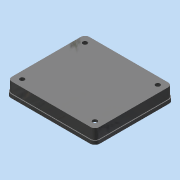
# Autodesk Inventor part: Plate
Saved by Autodesk Inventor 2012 (Build 160160000, 160)
## iProperties
Created: 2012-05-23
Part Number: Plate
Material: Default
Document SubType Name: Modeling
Designer: dgitz
Density: 1 g/cm^3
Author: dgitz
Autodesk Inventor part; units mm, degrees
ref_plane "YZ Plane" through (0, 0, 0) normal (1, 0, 0) x (0, 1, 0)
ref_plane "XZ Plane" through (0, 0, 0) normal (0, 1, 0) x (-1, 0, 0)
ref_plane "XY Plane" through (0, 0, 0) normal (0, 0, 1) x (1, 0, 0)
sketch "Sketch2" plane through (0, 0, 0) normal (0, 1, 0) x (-1, 0, 0)
  line L0 (-50.8, 50.8) -> (50.8, 50.8)
  line L1 (57.15, 44.45) -> (57.15, -44.45)
  line L2 (50.8, -50.8) -> (-50.8, -50.8)
  line L3 (-57.15, -44.45) -> (-57.15, 44.45)
  arc A0 (-50.8, 50.8) -> (-57.15, 44.45) centre (-50.8, 44.45) ccw
  arc A1 (-57.15, -44.45) -> (-50.8, -50.8) centre (-50.8, -44.45) ccw
  arc A2 (50.8, -50.8) -> (57.15, -44.45) centre (50.8, -44.45) ccw
  arc A3 (57.15, 44.45) -> (50.8, 50.8) centre (50.8, 44.45) ccw
  line L4 (50.8, 48.768) -> (-50.8, 48.768)
  arc A4 (-50.8, 48.768) -> (-55.118, 44.45) centre (-50.8, 44.45) ccw
  line L5 (-55.118, 44.45) -> (-55.118, -44.45)
  arc A5 (-55.118, -44.45) -> (-50.8, -48.768) centre (-50.8, -44.45) ccw
  line L6 (-50.8, -48.768) -> (50.8, -48.768)
  arc A6 (50.8, -48.768) -> (55.118, -44.45) centre (50.8, -44.45) ccw
  line L7 (55.118, -44.45) -> (55.118, 44.45)
  arc A7 (55.118, 44.45) -> (50.8, 48.768) centre (50.8, 44.45) ccw
  line L8 (-50.8, 44.45) -> (50.8, -44.45) construction
  point P0 (0, 0)
  point P1 (0, 0)
  point P2 (0, 0)
  dimension "d0" = 114.3
  dimension "d1" = 101.6
  dimension "d2" = 6.35
  dimension "d3" = 2.032
  constraints: 18 end point, 16 point on circle, 8 centre point, 8 tangent, 4 parallel, 3 equal radius, 2 coincident, 2 perpendicular, 1 horizontal, 1 midpoint, 7 other
  measures "d0" distance between parallel lines of L1 L3
  measures "d1" distance between parallel lines of L2 L0
  measures "d2" radius of A0
  measures "d3" distance between parallel lines of L5 L3
extrude "Extrusion1" add sketch "Sketch2" along normal blind 4.572
sketch "Sketch3" plane through (0, 4.572, 0) normal (0, 1, 0) x (1, 0, 0)
  line L0 (-55.118, -44.45) -> (-55.118, 44.45) projected
  arc A0 (-50.8, 48.768) -> (-55.118, 44.45) centre (-50.8, 44.45) ccw projected
  line L1 (-50.8, 48.768) -> (50.8, 48.768) projected
  line L2 (55.118, 44.45) -> (55.118, -44.45) projected
  line L3 (50.8, -48.768) -> (-50.8, -48.768) projected
  line L4 (-50.8, 49.784) -> (50.8, 49.784)
  line L5 (56.134, 44.45) -> (56.134, -44.45)
  line L6 (50.8, -49.784) -> (-50.8, -49.784)
  line L7 (-56.134, -44.45) -> (-56.134, 44.45)
  arc A1 (-50.8, 49.784) -> (-56.134, 44.45) centre (-50.8, 44.45) ccw
  arc A2 (-56.134, -44.45) -> (-50.8, -49.784) centre (-50.8, -44.45) ccw
  arc A3 (50.8, -49.784) -> (56.134, -44.45) centre (50.8, -44.45) ccw
  arc A4 (56.134, 44.45) -> (50.8, 49.784) centre (50.8, 44.45) ccw
  line L8 (-54.102, 44.45) -> (-54.102, -44.45)
  arc A5 (-54.102, -44.45) -> (-50.8, -47.752) centre (-50.8, -44.45) ccw
  line L9 (-50.8, -47.752) -> (50.8, -47.752)
  arc A6 (50.8, -47.752) -> (54.102, -44.45) centre (50.8, -44.45) ccw
  line L10 (54.102, -44.45) -> (54.102, 44.45)
  arc A7 (54.102, 44.45) -> (50.8, 47.752) centre (50.8, 44.45) ccw
  line L11 (50.8, 47.752) -> (-50.8, 47.752)
  arc A8 (-50.8, 47.752) -> (-54.102, 44.45) centre (-50.8, 44.45) ccw
  point P0 (0, 0)
  dimension "d7" = 1.016
  dimension "d8" = 1.016
  dimension "d9" = 1.016
  dimension "d10" = 1.016
  dimension "d11" = 2.032
  constraints: 16 end point, 16 point on circle, 8 centre point, 8 tangent, 4 parallel, 3 equal radius, 2 perpendicular, 1 concentric, 1 horizontal, 7 other
  measures "d7" distance between parallel lines of L7 L0
  measures "d8" distance between parallel lines of L4 L1
  measures "d9" distance between parallel lines of L5 L2
  measures "d10" distance between parallel lines of L3 L6
  measures "d11" distance between parallel lines of L8 L7
extrude "Extrusion2" add sketch "Sketch3" along normal blind 10.16
sketch "Sketch5" plane through (0, 14.732, 0) normal (0, 1, 0) x (1, 0, 0)
  arc A0 (-50.8, 49.784) -> (-56.134, 44.45) centre (-50.8, 44.45) ccw projected
  line L0 (-56.134, -44.45) -> (-56.134, 44.45) projected
  arc A1 (-56.134, -44.45) -> (-50.8, -49.784) centre (-50.8, -44.45) ccw projected
  line L1 (50.8, -49.784) -> (-50.8, -49.784) projected
  arc A2 (50.8, -49.784) -> (56.134, -44.45) centre (50.8, -44.45) ccw projected
  line L2 (56.134, 44.45) -> (56.134, -44.45) projected
  arc A3 (56.134, 44.45) -> (50.8, 49.784) centre (50.8, 44.45) ccw projected
  line L3 (-50.8, 49.784) -> (50.8, 49.784) projected
  point P0 (0, 0)
extrude "Extrusion3" add sketch "Sketch5" along normal blind 3.048
sketch "Sketch6" plane through (0, 17.78, 0) normal (0, 1, 0) x (1, 0, 0)
  line L0 (-50.8, 49.784) -> (50.8, 49.784) projected
  line L1 (-56.134, -44.45) -> (-56.134, 44.45) projected
  line L2 (56.134, 44.45) -> (56.134, -44.45) projected
  circle A0 centre (-46.736, 40.386) radius 2.921
  circle A1 centre (-46.736, -40.386) radius 2.921
  circle A2 centre (46.736, -40.386) radius 2.921
  circle A3 centre (46.736, 40.386) radius 2.921
  line L3 (-46.736, 40.386) -> (-46.736, -40.386) construction
  line L4 (-46.736, -40.386) -> (46.736, -40.386) construction
  line L5 (46.736, -40.386) -> (46.736, 40.386) construction
  line L6 (46.736, 40.386) -> (-46.736, 40.386) construction
  line L7 (-46.736, 40.386) -> (46.736, -40.386) construction
  point P0 (0, 0)
  point P1 (0, 0)
  dimension "d16" = 5.842
  dimension "d20" = 87.63
  dimension "d21" = 9.398
  dimension "d22" = 9.398
  constraints: 10 end point, 4 centre point, 3 equal radius, 2 parallel, 2 perpendicular, 1 coincident, 1 midpoint
  measures "d16" diameter of A0
  measures "d21" distance between parallel lines of L1 L3
  measures "d22" distance between parallel lines of L0 L6
extrude "Extrusion4" cut sketch "Sketch6" against normal through all
body "Solid1"
